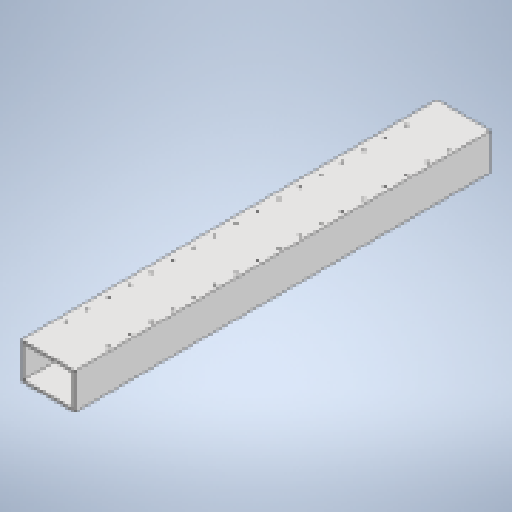
# Autodesk Inventor part: HORIZONTALTUBE
Saved by Autodesk Inventor 2023 (Build 270158000, 158)
## iProperties
Created: 2022-05-02
Part Number: HORIZONTALTUBE
Material: Generic
Document SubType Name: Modeling
Designer: plebbb
Density: 1 g/cm^3
Appearance: Default
Author: plebbb
Autodesk Inventor part; units mm, degrees
ref_plane "YZ Plane" through (0, 0, 0) normal (1, 0, 0) x (0, 1, 0)
ref_plane "XZ Plane" through (0, 0, 0) normal (0, 1, 0) x (-1, 0, 0)
ref_plane "XY Plane" through (0, 0, 0) normal (0, 0, 1) x (1, 0, 0)
sketch "Sketch1" plane through (0, 0, 0) normal (0, 0, 1) x (1, 0, 0)
  line L0 (0, 0) -> (152.4, 0)
  line L1 (152.4, 0) -> (152.4, 101.6)
  line L2 (152.4, 101.6) -> (0, 101.6)
  line L3 (0, 101.6) -> (0, 0)
  dimension "d0" = 152.4
  dimension "d1" = 101.6
  constraints: 8 end point, 2 parallel, 1 horizontal, 1 perpendicular
  measures "d0" distance of L1.end L2.end
  measures "d1" distance of L0.end L1.end
extrude "Extrusion1" add sketch "Sketch1" along normal blind 1174.2928
shell "Shell1" thickness 6.35 removed faces 2 at (50.8, 67.7333, 1174.2928) at (50.8, 67.7333, 0)
sketch "Sketch2" plane through (0, 101.6, 0) normal (0, 1, 0) x (1, 0, 0)
  circle A0 centre (127.4, -1067.1428) radius 3 projected
  circle A1 centre (127.4, -1007.1428) radius 3 projected
  circle A2 centre (127.4, -947.1428) radius 3 projected
  circle A3 centre (127.4, -887.1428) radius 3 projected
  circle A4 centre (127.4, -827.1428) radius 3 projected
  circle A5 centre (127.4, -767.1428) radius 3 projected
  circle A6 centre (127.4, -707.1428) radius 3 projected
  circle A7 centre (127.4, -647.1428) radius 3 projected
  circle A8 centre (127.4, -587.1428) radius 3 projected
  circle A9 centre (127.4, -527.1428) radius 3 projected
  circle A10 centre (127.4, -467.1428) radius 3 projected
  circle A11 centre (127.4, -407.1428) radius 3 projected
  circle A12 centre (127.4, -347.1428) radius 3 projected
  circle A13 centre (127.4, -287.1428) radius 3 projected
  circle A14 centre (127.4, -227.1428) radius 3 projected
  circle A15 centre (127.4, -167.1428) radius 3 projected
  circle A16 centre (127.4, -107.1428) radius 3 projected
  line L0 (117.4, -87.1428) -> (137.4, -87.1428) projected
  line L1 (137.4, -87.1428) -> (137.4, -1087.1428) projected
  line L2 (117.4, -1087.1428) -> (137.4, -1087.1428) projected
  line L3 (117.4, -87.1428) -> (117.4, -1087.1428) projected
  circle A17 centre (22.4, -1067.1428) radius 3 projected
  circle A18 centre (22.4, -1007.1428) radius 3 projected
  circle A19 centre (22.4, -947.1428) radius 3 projected
  circle A20 centre (22.4, -887.1428) radius 3 projected
  circle A21 centre (22.4, -827.1428) radius 3 projected
  circle A22 centre (22.4, -767.1428) radius 3 projected
  circle A23 centre (22.4, -707.1428) radius 3 projected
  circle A24 centre (22.4, -647.1428) radius 3 projected
  circle A25 centre (22.4, -587.1428) radius 3 projected
  circle A26 centre (22.4, -527.1428) radius 3 projected
  circle A27 centre (22.4, -467.1428) radius 3 projected
  circle A28 centre (22.4, -407.1428) radius 3 projected
  circle A29 centre (22.4, -347.1428) radius 3 projected
  circle A30 centre (22.4, -287.1428) radius 3 projected
  circle A31 centre (22.4, -227.1428) radius 3 projected
  circle A32 centre (22.4, -167.1428) radius 3 projected
  circle A33 centre (22.4, -107.1428) radius 3 projected
  line L4 (12.4, -87.1428) -> (32.4, -87.1428) projected
  line L5 (32.4, -87.1428) -> (32.4, -1087.1428) projected
  line L6 (12.4, -1087.1428) -> (32.4, -1087.1428) projected
  line L7 (12.4, -87.1428) -> (12.4, -1087.1428) projected
  point P0 (0, 0)
extrude "Extrusion2" cut sketch "Sketch2" against normal up to surface (6.35 mm away) contours A0 | A1 | A2 | A3 | A4 | A5 | A6 | A7 | A8 | A9 | A10 | A11 | A12 | A13 | A14 | A15 | A16 | A17 | A18 | A19 | A20 | A21 | A22 | A23 | A24 | A25 | A26 | A27 | A28 | A29 | A30 | A31 | A32 | A33
body "Solid1"
